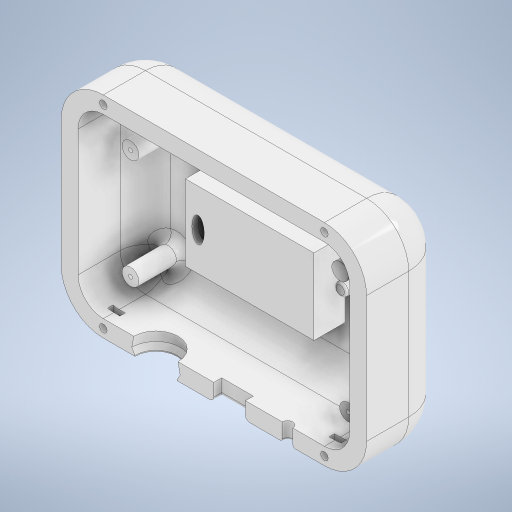
# Autodesk Inventor part: Case inferiore
Saved by Autodesk Inventor 2023 (Build 270158000, 158)
## iProperties
Created: 2022-12-30
Part Number: Case inferiore
Material: Plastica ABS
Document SubType Name: Modeling
Designer: Gabriele
Density: 1.06 g/cm^3
Appearance: Bianco
Author: Gabriele
Autodesk Inventor part; units mm, degrees
ref_plane "YZ Plane" through (0, 0, 0) normal (1, 0, 0) x (0, 1, 0)
ref_plane "XZ Plane" through (0, 0, 0) normal (0, 1, 0) x (-1, 0, 0)
ref_plane "XY Plane" through (0, 0, 0) normal (0, 0, 1) x (1, 0, 0)
sketch "Schizzo1" plane through (0, 0, 0) normal (0, 0, 1) x (1, 0, 0)
  line L0 (-52.5, -50) -> (52.5, -50)
  line L1 (72.5, -30) -> (72.5, 30)
  line L2 (52.5, 50) -> (-52.5, 50)
  line L3 (-72.5, 30) -> (-72.5, -30)
  line L4 (-72.5, -50) -> (72.5, 50) construction
  line L5 (72.5, -50) -> (-72.5, 50) construction
  arc A0 (-52.5, 50) -> (-72.5, 30) centre (-52.5, 30) ccw
  arc A1 (-72.5, -30) -> (-52.5, -50) centre (-52.5, -30) ccw
  arc A2 (52.5, -50) -> (72.5, -30) centre (52.5, -30) ccw
  arc A3 (72.5, 30) -> (52.5, 50) centre (52.5, 30) ccw
  point P0 (0, 0)
  dimension "d0" = 145
  dimension "d1" = 100
  dimension "d2" = 20
  constraints: 12 end point, 8 point on circle, 8 point on line, 8 tangent, 4 centre point, 3 equal radius, 2 midpoint, 2 parallel, 1 horizontal, 1 perpendicular
  measures "d0" distance of L4.end L5.end
  measures "d1" distance of L5.end L4.start
  measures "d2" radius of A0
extrude "Estrusione1" add sketch "Schizzo1" along normal blind 40
fillet "Raccordo1" radius 20 8 edges at (-66.6421, 44.1421, 0) (-72.5, 0, 0) (-66.6421, -44.1421, 0) (0, -50, 0) (66.6421, -44.1421, 0) (72.5, 0, 0) (66.6421, 44.1421, 0) (0, 50, 0)
shell "Svuotamento1" thickness 8 removed faces 1 at (17.5, -16.6667, 40)
sketch "Schizzo4" plane through (-52.5, -50, 40) normal (0, -1, 0) x (1, 0, 0)
  line L0 (52.5, -3.75) -> (67.5, -3.75)
  line L1 (67.5, -3.75) -> (67.5, 3.75)
  line L2 (67.5, 3.75) -> (52.5, 3.75)
  line L3 (52.5, 3.75) -> (52.5, -3.75)
  line L4 (0, 0) -> (105, 0) projected
  line L5 (52.5, -3.75) -> (67.5, 3.75) construction
  line L6 (67.5, -3.75) -> (52.5, 3.75) construction
  circle A0 centre (25, 0) radius 10
  circle A1 centre (87.5, 0) radius 2.55
  line L7 (105, -20) -> (105, 0) projected
  point P0 (52.5, -40)
  point P1 (52.5, 0)
  point P2 (90.05, 0)
  point P3 (84.95, 0)
  point P4 (35, 0)
  point P5 (15, 0)
  point P6 (52.5, 0)
  point P7 (52.5, 0)
  dimension "d8" = 15
  dimension "d9" = 7.5
  dimension "d10" = 20
  dimension "d11" = 5.1
  dimension "d18" = 3.75
  dimension "d107" = 25
  dimension "d113" = 17.5
  dimension "d114" = 27.5
  constraints: 12 end point, 3 midpoint, 2 centre point, 2 parallel, 2 point on line, 1 horizontal, 1 perpendicular
  measures "d8" distance of L1.end L2.end
  measures "d9" distance of L0.end L1.end
  measures "d10" diameter of A0
  measures "d11" diameter of A1
  measures "d18" distance from line of L4 L0.start
  measures "d107" distance of L4.start A0.centre
  measures "d113" distance from line of L7 A1.centre
  measures "d114" distance from line of L3 A0.centre
extrude "Estrusione2" cut sketch "Schizzo4" against normal blind 9 contours L3 L4 L1 L0 | L3 L2 L1 L4 | L4 A0 | L4 A1 picked at (23.1065, -2.7433) picked at (86.6747, -0.2034)
sketch "Schizzo6" plane through (0, 0, 40) normal (0, 0, 1) x (1, 0, 0)
  circle A0 centre (-52.5, 46) radius 1.8
  circle A1 centre (52.5, 46) radius 1.8
  line L0 (52.5, -30) -> (52.5, -50) projected
  circle A2 centre (52.5, -46) radius 1.8
  line L1 (-52.5, -50) -> (-52.5, -30) projected
  circle A3 centre (-52.5, -46) radius 1.8
  line L2 (-72.5, 30) -> (-72.5, -30) projected
  line L3 (-52.5, -50) -> (52.5, -50) projected
  line L4 (-52.5, -50) -> (52.5, -50) projected
  line L5 (52.5, 50) -> (-52.5, 50) projected
  point P0 (0, 0)
  point P1 (32.45, -50)
  point P2 (-17.5, -50)
  dimension "d19" = 3.6
  dimension "d20" = 3.6
  dimension "d21" = 3.6
  dimension "d22" = 3.6
  dimension "d23" = 20
  dimension "d24" = 4
  dimension "d25" = 4
  dimension "d26" = 4
  dimension "d27" = 4
  constraints: 4 centre point, 2 point on line
  measures "d19" diameter of A0
  measures "d20" diameter of A1
  measures "d21" diameter of A2
  measures "d22" diameter of A3
  measures "d23" distance from line of L2 A0.centre
  measures "d24" distance from line of L3 A3.centre
  measures "d25" distance from line of L4 A2.centre
  measures "d26" distance from line of L5 A0.centre
  measures "d27" distance from line of L5 A1.centre
extrude "Estrusione3" cut sketch "Schizzo6" against normal blind 18
sketch "Schizzo8" plane through (-52.5, 42, 20) normal (0, -1, 0) x (1, 0, 0)
  line L0 (-2.9, 12.5) -> (2.9, 12.5)
  line L1 (2.9, 12.5) -> (2.9, 15)
  line L2 (2.9, 15) -> (-2.9, 15)
  line L3 (-2.9, 15) -> (-2.9, 12.5)
  line L4 (0, 0) -> (0, 20) projected
  line L5 (-2.9, 12.5) -> (2.9, 15) construction
  line L6 (2.9, 12.5) -> (-2.9, 15) construction
  line L7 (0, 20) -> (105, 20) projected
  line L8 (102.1, 12.5) -> (107.9, 12.5)
  line L9 (107.9, 12.5) -> (107.9, 15)
  line L10 (107.9, 15) -> (102.1, 15)
  line L11 (102.1, 15) -> (102.1, 12.5)
  line L12 (105, 0) -> (105, 20) projected
  line L13 (102.1, 12.5) -> (107.9, 15) construction
  line L14 (107.9, 12.5) -> (102.1, 15) construction
  point P0 (52.5, -20)
  point P1 (0, 13.75)
  point P2 (105, 13.75)
  dimension "d30" = 2.5
  dimension "d31" = 5.8
  dimension "d32" = 5
  dimension "d33" = 5.8
  dimension "d34" = 2.5
  dimension "d35" = 5
  constraints: 24 end point, 4 midpoint, 4 parallel, 2 horizontal, 2 perpendicular, 2 point on line
  measures "d30" distance of L0.end L1.end
  measures "d31" distance of L1.end L2.end
  measures "d32" distance between parallel lines of L7 L2
  measures "d33" distance of L9.end L10.end
  measures "d34" distance of L10.end L8.start
  measures "d35" distance between parallel lines of L7 L10
extrude "Estrusione4" cut sketch "Schizzo8" along normal blind 2 and the other way blind 7.1
sketch "Schizzo9" plane through (52.5, -42, 40) normal (0, 1, 0) x (1, 0, 0)
  line L0 (3.05, 7.5) -> (-2.75, 7.5)
  line L1 (-2.75, 7.5) -> (-2.75, 5)
  line L2 (-2.75, 5) -> (3.05, 5)
  line L3 (3.05, 5) -> (3.05, 7.5)
  line L4 (0, 20) -> (0, 0) projected
  line L5 (3.05, 7.5) -> (-2.75, 5) construction
  line L6 (-2.75, 7.5) -> (3.05, 5) construction
  line L7 (-102.1, 7.5) -> (-107.9, 7.5)
  line L8 (-107.9, 7.5) -> (-107.9, 5)
  line L9 (-107.9, 5) -> (-102.1, 5)
  line L10 (-102.1, 5) -> (-102.1, 7.5)
  line L11 (-105, 20) -> (-105, 0) projected
  line L12 (-102.1, 7.5) -> (-107.9, 5) construction
  line L13 (-107.9, 7.5) -> (-102.1, 5) construction
  line L14 (0, 0) -> (-105, 0) projected
  line L15 (0, 0) -> (-105, 0) projected
  point P0 (-52.5, 40)
  point P1 (-105, 6.25)
  point P2 (-70, 0)
  point P3 (-20.05, 0)
  dimension "d40" = 5.8
  dimension "d41" = 2.5
  dimension "d42" = 5
  dimension "d43" = 2.75
  dimension "d44" = 5
  dimension "d45" = 2.5
  dimension "d46" = 5.8
  constraints: 24 end point, 4 parallel, 2 horizontal, 2 midpoint, 2 perpendicular, 1 point on line
  measures "d40" distance of L1.end L2.end
  measures "d41" distance of L0.end L1.end
  measures "d42" distance between parallel lines of L14 L2
  measures "d43" distance between parallel lines of L4 L1
  measures "d44" distance between parallel lines of L15 L9
  measures "d45" distance of L9.end L7.start
  measures "d46" distance of L7.start L7.end
extrude "Estrusione5" cut sketch "Schizzo9" along normal blind 2 and the other way blind 7.1
sketch "Schizzo10" plane through (0, 0, 0) normal (0, 0, -1) x (-1, 0, 0)
  line L0 (27.5, 15) -> (-27.5, 15)
  line L1 (-27.5, 15) -> (-27.5, -15)
  line L2 (-27.5, -15) -> (27.5, -15)
  line L3 (27.5, -15) -> (27.5, 15)
  line L4 (27.5, 15) -> (-27.5, -15) construction
  line L5 (-27.5, 15) -> (27.5, -15) construction
  point P0 (0, 0)
  dimension "d51" = 55
  dimension "d52" = 30
  constraints: 12 end point, 2 midpoint, 2 parallel, 1 horizontal, 1 perpendicular
  measures "d51" distance of L1.end L2.end
  measures "d52" distance of L0.end L1.end
extrude "Estrusione6" cut sketch "Schizzo10" against normal blind 20
sketch "Schizzo12" plane through (0, 0, 0) normal (0, 0, -1) x (-1, 0, 0)
  line L0 (30.5, 18) -> (-30.5, 18)
  line L1 (-30.5, -18) -> (30.5, -18)
  line L2 (30.5, 18) -> (-30.5, -18) construction
  line L3 (-30.5, 18) -> (30.5, -18) construction
  line L4 (30.5, -4) -> (38.5, -4)
  line L5 (38.5, -4) -> (38.5, 4)
  line L6 (38.5, 4) -> (30.5, 4)
  line L7 (30.5, -18) -> (30.5, -4)
  line L8 (30.5, 4) -> (30.5, 18)
  line L9 (-30.5, -4) -> (-38.5, -4)
  line L10 (-38.5, -4) -> (-38.5, 4)
  line L11 (-38.5, 4) -> (-30.5, 4)
  line L12 (-30.5, 18) -> (-30.5, 4)
  line L13 (-30.5, -4) -> (-30.5, -18)
  point P0 (0, 0)
  dimension "d60" = 61
  dimension "d61" = 36
  dimension "d62" = 8
  dimension "d63" = 8
  dimension "d64" = 4
  dimension "d65" = 8
  dimension "d66" = 8
  dimension "d67" = 4
  dimension "d68" = 8
  constraints: 28 end point, 8 perpendicular, 5 parallel, 3 horizontal, 2 midpoint
  measures "d60" distance of L1.start L1.end
  measures "d61" distance of L0.end L1.start
  measures "d62" distance of L5.end L6.end
  measures "d63" distance of L4.end L5.end
  measures "d64" distance from line of L6 point (0, 0)
  measures "d65" distance of L10.end L11.end
  measures "d66" distance of L9.end L10.end
  measures "d67" distance from line of point (0, 0) L11
  measures "d68" distance of L4.start L4.end
extrude "Estrusione8" cut sketch "Schizzo12" against normal blind 2
sketch "Schizzo11" plane through (-52.5, 30, 8) normal (0, 0, 1) x (1, 0, 0)
  line L0 (22, -48) -> (83, -48)
  line L1 (83, -48) -> (83, -12)
  line L2 (83, -12) -> (22, -12)
  line L3 (22, -12) -> (22, -48)
  line L4 (22, -48) -> (83, -12) construction
  line L5 (83, -48) -> (22, -12) construction
  point P0 (52.5, -30)
  dimension "d55" = 61
  dimension "d56" = 36
  constraints: 12 end point, 2 midpoint, 2 parallel, 1 horizontal, 1 perpendicular
  measures "d55" distance of L1.end L2.end
  measures "d56" distance of L0.end L1.end
extrude "Estrusione7" add sketch "Schizzo11" along normal blind 15
sketch "Schizzo15" plane through (0, 0, 2) normal (0, 0, -1) x (-1, 0, 0)
  line L0 (-30.5, -4) -> (-38.5, -4) projected
  line L1 (38.5, -4) -> (30.5, -4) projected
  point P0 (0, 0)
  point P1 (34, 0)
  point P2 (-34, 0)
  dimension "d78" = 34
  dimension "d79" = 34
  dimension "d80" = 4
  dimension "d81" = 4
  measures "d78" distance of point (0, 0) point (34, 0)
  measures "d79" distance of point (0, 0) point (-34, 0)
  measures "d80" distance from line of L0 point (-34, 0)
  measures "d81" distance from line of L1 point (34, 0)
hole "Foro1" at (-34, 0, 2) at (34, 0, 2) direction (0, 0, 1) diameter 1.8 depth 5
fillet "Raccordo2" radius 2 3 edges at (0, -50, 38.125) (7.5, -50, 36.25) (15, -50, 38.125)
fillet "Raccordo3" radius 1 1 edges at (35, -50, 37.45)
sketch "Schizzo21" plane through (-52.5, 30, 8) normal (0, 0, 1) x (1, 0, 0)
  circle A0 centre (2.7, -6.5) radius 4
  line L0 (105, 0) -> (0, 0) projected
  line L1 (0, 0) -> (0, -60) projected
  line L2 (105, -60) -> (105, 0) projected
  line L3 (0, 12) -> (105, 12) projected
  line L4 (-12, -60) -> (-12, 0) projected
  circle A1 centre (2.7, -58.5) radius 4
  line L5 (15, -72) -> (0, -72) projected
  circle A2 centre (106, -62.5) radius 4
  line L6 (117, 0) -> (117, -60) projected
  line L7 (105, -72) -> (90.05, -72) projected
  circle A3 centre (102.3, -6.5) radius 4
  point P0 (52.5, -30)
  point P1 (0, -3.5487)
  point P2 (0, -9.4513)
  point P3 (0, -59.8077)
  point P4 (0, -55.5487)
  dimension "d117" = 8
  dimension "d139" = 18.5
  dimension "d140" = 14.7
  dimension "d141" = 8
  dimension "d142" = 14.7
  dimension "d143" = 13.5
  dimension "d144" = 8
  dimension "d145" = 11
  dimension "d146" = 9.5
  dimension "d148" = 8
  dimension "d149" = 14.7
  dimension "d150" = 18.5
  constraints: 4 centre point
  measures "d117" diameter of A0
  measures "d139" distance from line of L3 A0.centre
  measures "d140" distance from line of L4 A0.centre
  measures "d141" diameter of A1
  measures "d142" distance from line of L4 A1.centre
  measures "d143" distance from line of L5 A1.centre
  measures "d144" diameter of A2
  measures "d145" distance from line of L6 A2.centre
  measures "d146" distance from line of L7 A2.centre
  measures "d148" diameter of A3
  measures "d149" distance from line of L6 A3.centre
  measures "d150" distance from line of L3 A3.centre
extrude "Estrusione12" add sketch "Schizzo21" along normal blind 21.8
sketch "Schizzo23" plane through (0, 0, 40) normal (0, 0, 1) x (1, 0, 0)
  line L0 (-16, -47) -> (-18.5, -34.5) projected
  line L1 (-17.75, -50) -> (-16, -47) projected
  line L2 (0, -42) -> (-17.5, -42) projected
  line L3 (-17, -42) -> (-27.5, -42)
  line L4 (52.5, -42) -> (-52.5, -42) projected
  line L5 (-17.75, -50) -> (-27.5, -50)
  line L6 (-17.5, -50) -> (-37.5, -50) projected
  line L7 (-27.5, -50) -> (-27.5, -42)
  line L8 (-17, -42) -> (-16, -47)
  line L9 (-17.75, -50) -> (-16, -47)
  point P0 (0, 0)
  constraints: 10 end point, 3 point on line, 1 collinear, 1 midpoint, 1 perpendicular
revolve "Rivoluzione1" cut sketch "Schizzo23" angle 360 about axis through (-27.5, -50, 40) along (0, 1, 0)
sketch "Schizzo24" plane through (-49.8, 23.5, 29.8) normal (0, 0, 1) x (1, 0, 0)
  arc A0 (-2.7, -2.9513) -> (-2.7, 2.9513) centre (0, 0) ccw projected
  circle A1 centre (0, 0) radius 0.95
  circle A2 centre (0, -52) radius 4 projected
  circle A3 centre (0, -52) radius 0.95
  circle A4 centre (103.3, -56) radius 4 projected
  circle A5 centre (103.3, -56) radius 0.95
  point P0 (49.8, -23.5)
  point P1 (85, 0)
  point P2 (0, -50)
  point P3 (85, -50)
  dimension "d133" = 1.9
  dimension "d147" = 1.9
  dimension "d159" = 1.9
  constraints: 3 centre point, 3 coincident
  measures "d133" diameter of A1
  measures "d147" diameter of A5
  measures "d159" diameter of A3
extrude "Estrusione13" cut sketch "Schizzo24" against normal blind 10 contours A1 | A3 | A5
sketch "Schizzo25" plane through (-52.5, 30, 8) normal (0, 0, -1) x (-1, 0, 0)
  line L0 (-80, -45) -> (-25, -45) projected
  line L1 (-25, -45) -> (-25, -15) projected
  line L2 (-25, -15) -> (-80, -15) projected
  line L3 (-80, -15) -> (-80, -45) projected
  point P0 (-52.5, -30)
extrude "Estrusione14" cut sketch "Schizzo25" against normal blind 12
sketch "Schizzo26" plane through (-52.5, 30, 23) normal (0, 0, 1) x (1, 0, 0)
  ellipse E0 centre (28, -30) end of major axis (28, -24) minor radius 2.9368
  line L0 (22, -12) -> (22, -48) projected
  point P0 (52.5, -30)
  dimension "d157" = 6
  dimension "d158" = 6
  constraints: 2 other
  measures "d158" distance from line of L0 point (28, -30)
extrude "Estrusione15" cut sketch "Schizzo26" against normal blind 12
sketch "Schizzo27" plane through (-52.5, 30, 8) normal (0, 0, 1) x (1, 0, 0)
  circle A0 centre (86.5, -30) radius 0.9 projected
  circle A1 centre (18.5, -30) radius 0.9 projected
  circle A2 centre (18.5, -30) radius 0.9 projected
  circle A3 centre (86.5, -30) radius 0.9 projected
  circle A4 centre (18.5, -30) radius 3
  circle A5 centre (86.5, -30) radius 3
  point P0 (52.5, -30)
  dimension "d160" = 6
  dimension "d161" = 6
  constraints: 2 centre point, 2 coincident
  measures "d160" diameter of A4
  measures "d161" diameter of A5
extrude "Estrusione16" add sketch "Schizzo27" along normal blind 6 contours A0 | A1 | A4 | A5
fillet "Raccordo4" radius 1 1 edges at (31, 0, 14)
fillet "Raccordo5" radius 1 1 edges at (-37, 0, 14)
sketch "Schizzo28" plane through (34, 0, 7) normal (0, 0, -1) x (-1, 0, 0)
  circle A0 centre (0, 0) radius 0.9 projected
  circle A1 centre (68, 0) radius 0.9 projected
  point P0 (34, 0)
extrude "Estrusione17" cut sketch "Schizzo28" against normal blind 4
fillet "Raccordo9" radius 2 1 edges at (-37, 0, 8)
fillet "Raccordo10" radius 2 1 edges at (31, 0, 8)
fillet "Raccordo11" radius 4 3 edges at (-53.8, 23.5002, 8.0706) (-48.1875, 27.1606, 8) (-48.1875, 19.8394, 8)
fillet "Raccordo12" radius 4 8 edges at (45.8, 23.5, 8) (53.4857, 25.0543, 8.0405) (53.4857, 21.9457, 8.0405) (-49.0683, -32.4325, 8.2491) (-53.1205, -30.7304, 8.0383) (-53.7164, -27.6863, 8.0618) (-48.1875, -24.8394, 8) (-45.8737, -29.2641, 8)
fillet "Raccordo13" radius 2 5 edges at (51.3274, -29.1414, 8) (54.9263, -28.7629, 8.2478) (57.2741, -31.1747, 9.0534) (55.9818, -35.637, 9.9949) (49.841, -34.116, 8.728)
